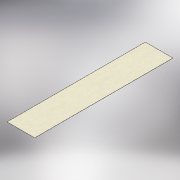
# Autodesk Inventor part: Bande
Saved by Autodesk Inventor 2017 (Build 210142000, 142)
## iProperties
Part Number: Bande
Material: Papier
Document SubType Name: Modeling
Designer: Adrien MARY
Mass: 1.488 g
Surface Area: 160.96 cm^2
Volume: 1.6 cm^3
Density: 0.93 g/cm^3
Appearance: Carton - Panneau de particules
Stock Number: 1440-01-04
Author: Adrien MARY
Autodesk Inventor part; units mm, degrees
ref_plane "YZ Plane" through (0, 0, 0) normal (1, 0, 0) x (0, 1, 0)
ref_plane "XZ Plane" through (0, 0, 0) normal (0, 1, 0) x (-1, 0, 0)
ref_plane "XY Plane" through (0, 0, 0) normal (0, 0, 1) x (1, 0, 0)
sketch "Esquisse1" plane through (0, 0, 0) normal (0, 0, 1) x (1, 0, 0)
  line L0 (-20, 0) -> (20, 0)
  line L1 (20, 0) -> (20, 200)
  line L2 (20, 200) -> (-20, 200)
  line L3 (-20, 200) -> (-20, 0)
  point P0 (0, 0)
  point P1 (0, 0)
  dimension "d0" = 40
  dimension "d1" = 200
  constraints: 8 end point, 2 parallel, 1 coincident, 1 horizontal, 1 midpoint, 1 perpendicular
  measures "d0" distance of L0.start L0.end
  measures "d1" distance of L0.end L1.end
extrude "Extrusion1" add sketch "Esquisse1" along normal blind 0.2
